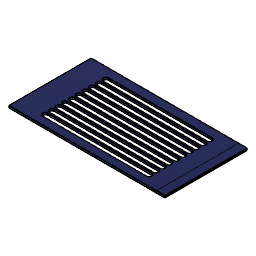
back_dynamic_wall (Autodesk Fusion 360 design; units mm, degrees)
part number: 2026-07-10-05-34-35-555
Autodesk Fusion 360 part; units mm, degrees
sketch "Sketch1" plane through (0, 0, 0) normal (0, 0, 1) x (1, 0, 0)
  line L0 (0, 0) -> (180, 0)
  line L1 (180, 0) -> (180, 95)
  line L2 (180, 95) -> (0, 95)
  line L3 (0, 95) -> (0, 0)
  dimension "d1" = 95
  dimension "d2" = 180
  constraint horizontal L0
  constraint vertical L1
  constraint horizontal L2
  constraint vertical L3
  constraint coincident L0.start L3.end
  measures "d1" distance of L0.start L2.end
  measures "d2" distance of L1.end L2.end
extrude "Extrude1" add sketch "Sketch1" along normal blind 2.5
sketch "Sketch2" plane through (0, 0, 2.5) normal (0, 0, 1) x (-1, 0, 0)
  line L0 (0, -95) -> (0, 0)
  line L1 (0, 0) -> (-180, 0)
  line L2 (-180, 0) -> (-180, -95)
  line L3 (-180, -95) -> (0, -95)
  line L4 (-30, -85) -> (-150, -85)
  line L5 (-150, -79) -> (-30, -79)
  arc A0 (-150, -79) -> (-150, -85) centre (-150, -82) ccw
  arc A1 (-30, -85) -> (-30, -79) centre (-30, -82) ccw
  dimension "d5" = 6
  dimension "d6" = 120
  dimension "d7" = 6
  dimension "d8" = 10
  dimension "d14" = 30
  constraint horizontal L4
  constraint horizontal L5
  measures "d5" distance of L4.end L5.start
  measures "d6" distance of L5.start L5.end
  measures "d7" diameter of A0
  measures "d8" distance of L3 L4
  measures "d14" distance of L0 A1.centre
extrude "Extrude2" cut sketch "Sketch2" against normal through all contours L4 L5 A0 A1
pattern_linear "R-Pattern1" count 1 spacing 0 along (1, 0, 0) count 10 spacing 7.7778 along (0, -1, 0) of "Extrude2"
hole "Hole1" at (180, 1.7635, 1.2997) direction (-1, 0, 0) diameter 1.5 depth 10 tip angle 180
pattern_linear "R-Pattern2" count 1 spacing 2 along (0, 0, -1) count 50 spacing 1.8776 along (0, 1, 0) of "Hole1"
